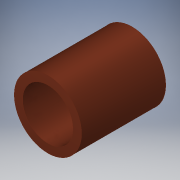
# Autodesk Inventor part: coil
Saved by Autodesk Inventor 2019 (Build 230136000, 136)
## iProperties
Created: 2021-07-12
Part Number: coil
Material: Generic
Document SubType Name: Modeling
Designer: pensun
Density: 1 g/cm^3
Appearance: Default
Author: pensun
Autodesk Inventor part; units mm, degrees
ref_plane "YZ Plane" through (0, 0, 0) normal (1, 0, 0) x (0, 1, 0)
ref_plane "XZ Plane" through (0, 0, 0) normal (0, 1, 0) x (-1, 0, 0)
ref_plane "XY Plane" through (0, 0, 0) normal (0, 0, 1) x (1, 0, 0)
sketch "Sketch1" plane through (0, 0, 0) normal (0, 0, 1) x (1, 0, 0)
  circle A0 centre (0, 0) radius 15
  circle A1 centre (0, 0) radius 20
  dimension "d0" = 0
  dimension "d1" = 0
  dimension "d2" = 30
  dimension "d3" = 0
  dimension "d4" = 0
  dimension "d5" = 40
  constraints: 2 centre point
  measures "d0" distance of point (0, 0) A0.centre
  measures "d1" distance of point (0, 0) A0.centre
  measures "d2" diameter of A0
  measures "d3" distance of point (0, 0) A1.centre
  measures "d4" distance of point (0, 0) A1.centre
  measures "d5" diameter of A1
extrude "Extrusion1" add sketch "Sketch1" along normal blind 50
body "Solid1"
